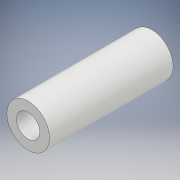
# Autodesk Inventor part: tuleja18
Saved by Autodesk Inventor 2017 (Build 210142000, 142)
## iProperties
Created: 2017-05-09
Part Number: tuleja18
Material: PCW, nieplastyfikowany
Document SubType Name: Modeling
Designer: Damian
Density: 1.29 g/cm^3
Appearance: Gładki - biały
Mass: 0.490209 g
Surface Area: 5.8509 cm^2
Volume: 0.380007 cm^3
Author: Damian
Autodesk Inventor part; units mm, degrees
ref_plane "YZ Plane" through (0, 0, 0) normal (1, 0, 0) x (0, 1, 0)
ref_plane "XZ Plane" through (0, 0, 0) normal (0, 1, 0) x (-1, 0, 0)
ref_plane "XY Plane" through (0, 0, 0) normal (0, 0, 1) x (1, 0, 0)
sketch "Szkic1" plane through (0, 0, 0) normal (0, 1, 0) x (-1, 0, 0)
  circle A0 centre (0, 0) radius 1.7
  circle A1 centre (0, 0) radius 3.1
  dimension "d0" = 3.4
  dimension "d1" = 6.2
  constraints: 2 centre point, 2 coincident
  measures "d0" diameter of A0
  measures "d1" diameter of A1
extrude "Wyciągnięcie proste1" add sketch "Szkic1" along normal blind 18
